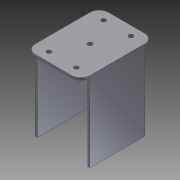
# Autodesk Inventor part: Caster2
Saved by Autodesk Inventor 2012 (Build 160160000, 160)
## iProperties
Created: 2011-10-20
Part Number: Caster2
Material: Default
Document SubType Name: Modeling
Designer: robotics
Density: 1 g/cm^3
Author: robotics
Autodesk Inventor part; units mm, degrees
ref_plane "YZ Plane" through (0, 0, 0) normal (1, 0, 0) x (0, 1, 0)
ref_plane "XZ Plane" through (0, 0, 0) normal (0, 1, 0) x (-1, 0, 0)
ref_plane "XY Plane" through (0, 0, 0) normal (0, 0, 1) x (1, 0, 0)
sketch "Sketch2" plane through (0, 0, 0) normal (0, 1, 0) x (-1, 0, 0)
  line L0 (-38.1, 50.8) -> (38.1, 50.8)
  line L1 (38.1, 50.8) -> (38.1, -50.8)
  line L2 (38.1, -50.8) -> (-38.1, -50.8)
  line L3 (-38.1, -50.8) -> (-38.1, 50.8)
  point P0 (0, 0)
  dimension "d0" = 38.1
  dimension "d1" = 38.1
  dimension "d2" = 50.8
  dimension "d3" = 50.8
  constraints: 8 end point, 2 parallel, 1 horizontal, 1 perpendicular
  measures "d0" distance from line of L1 point (0, 0)
  measures "d1" distance from line of L3 point (0, 0)
  measures "d2" distance from line of L0 point (0, 0)
  measures "d3" distance from line of L2 point (0, 0)
extrude "Extrusion1" add sketch "Sketch2" along normal blind 3.175
fillet "Fillet1" radius 12.7 4 edges at (38.1, 1.5875, 50.8) (-38.1, 1.5875, 50.8) (38.1, 1.5875, -50.8) (-38.1, 1.5875, -50.8)
sketch "Sketch3" plane through (0, 3.175, 0) normal (0, 1, 0) x (1, 0, 0)
  line L0 (-38.1, -38.1) -> (-38.1, 38.1) projected
  line L1 (25.4, -50.8) -> (-25.4, -50.8) projected
  line L2 (38.1, 38.1) -> (38.1, -38.1) projected
  line L3 (-25.4, 50.8) -> (25.4, 50.8) projected
  point P0 (0, 0)
  point P1 (-19.05, 38.1)
  point P2 (19.05, 38.1)
  point P3 (19.05, -38.1)
  point P4 (-19.05, -38.1)
  point P5 (0, 0)
  dimension "d7" = 12.7
  dimension "d8" = 19.05
  dimension "d9" = 19.05
  dimension "d10" = 12.7
  constraints: 2 horizontal alignment, 2 vertical alignment, 1 coincident
  measures "d7" distance from line of L3 point (-19.05, 38.1)
  measures "d8" distance from line of L0 point (-19.05, 38.1)
  measures "d9" distance from line of L2 point (19.05, 38.1)
  measures "d10" distance from line of L1 point (-19.05, -38.1)
hole "Hole1" at (-19.05, 3.175, -38.1) at (19.05, 3.175, -38.1) at (19.05, 3.175, 38.1) at (-19.05, 3.175, 38.1) at (0, 3.175, 0) direction (0, -1, 0) diameter 6.35 end through all
sketch "Sketch4" plane through (0, 0, 0) normal (0, -1, 0) x (1, 0, 0)
  circle A0 centre (-19.05, 38.1) radius 3.175 projected
  line L0 (38.1, -38.1) -> (38.1, 38.1) projected
  line L1 (-38.1, 38.1) -> (-38.1, -38.1) projected
  line L2 (38.1, 38.1) -> (34.925, 38.1)
  line L3 (34.925, 38.1) -> (34.925, -38.1)
  line L4 (34.925, -38.1) -> (38.1, -38.1)
  line L5 (38.1, -38.1) -> (38.1, 38.1)
  line L6 (-38.1, 38.1) -> (-34.925, 38.1)
  line L7 (-34.925, 38.1) -> (-34.925, -38.1)
  line L8 (-34.925, -38.1) -> (-38.1, -38.1)
  line L9 (-38.1, -38.1) -> (-38.1, 38.1)
  dimension "d18" = 3.175
  dimension "d19" = 3.175
  dimension "d20" = 76.2
  dimension "d21" = 76.2
  constraints: 16 end point, 4 parallel, 2 horizontal, 2 horizontal alignment, 2 perpendicular, 2 point on line
  measures "d18" distance of L6.start L6.end
  measures "d19" distance of L2.start L2.end
  measures "d20" distance of L2.end L3.end
  measures "d21" distance of L6.end L7.end
extrude "Extrusion2" add sketch "Sketch4" along normal blind 107.95 contours L4 L3 L2 L0 | L6 L7 L8 L1
equation "\"d1\" = d0"
equation "\"d3\" = d2"
equation "\"d4\" = metalThickness"
equation "\"d18\" = metalThickness"
equation "\"d19\" = metalThickness"
equation "\"d21\" = d20"
equation "\"metalThickness\" = 3.175"
body "Solid1"
